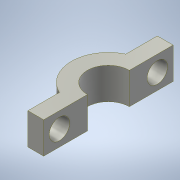
# Autodesk Inventor part: держатель
Saved by Autodesk Inventor 2021 (Build 250183000, 183)
## iProperties
Created: 2023-02-18
Part Number: держатель
Material: Типовые
Document SubType Name: Modeling
Designer: Tasya
Density: 1 g/cm^3
Appearance: Гладкий - слоновая кость
Author: Tasya
Autodesk Inventor part; units mm, degrees
ref_plane "YZ Plane" through (0, 0, 0) normal (1, 0, 0) x (0, 1, 0)
ref_plane "XZ Plane" through (0, 0, 0) normal (0, 1, 0) x (-1, 0, 0)
ref_plane "XY Plane" through (0, 0, 0) normal (0, 0, 1) x (1, 0, 0)
sketch "Эскиз1" plane through (0, 0, 0) normal (0, 1, 0) x (-1, 0, 0)
  line L0 (0, 12.3246) -> (0, 4)
  line L1 (0, 12.3246) -> (3, 12.3246)
  line L2 (3, 12.3246) -> (3, 6.3246)
  arc A0 (4, 0) -> (0, 4) centre (0, 0) ccw
  arc A1 (7, 0) -> (3, 6.3246) centre (0, 0) ccw
  line L3 (7, 0) -> (4, 0)
  line L4 (0, 0) -> (0, -3.8949) construction
  line L5 (0, 0) -> (4, 0) construction
  dimension "d0" = 4
  dimension "d1" = 7
  dimension "d2" = 6
  dimension "d3" = 3
  constraints: 12 end point, 4 point on circle, 3 horizontal, 2 centre point, 2 coincident, 2 collinear, 2 vertical, 1 perpendicular
  measures "d0" radius of A0
  measures "d1" radius of A1
  measures "d2" distance of L1.end L2.end
  measures "d3" distance of L0.start L1.end
extrude "Выдавливание1" add sketch "Эскиз1" along normal mid plane 6
sketch "Эскиз2" plane through (-3, -3, 12.3246) normal (-1, 0, 0) x (0, 0, 1)
  line L0 (0, 0) -> (0, 6) projected
  line L1 (-6, 6) -> (0, 6) projected
  line L2 (-6, 0) -> (-6, 6) projected
  line L3 (0, 0) -> (-6, 0) projected
  line L4 (0, 0) -> (-6, 6) construction
  line L5 (0, 6) -> (-8.3246, 6) construction
  line L6 (0, 6) -> (-6, 0) construction
  point P0 (-12.3246, 3)
  point P1 (-3, 3)
  constraints: 4 end point, 1 midpoint, 1 perpendicular
hole "Отверстие1" at (-3, 0, 9.3246) direction (1, 0, 0) diameter 3.9 end through all
mirror "Зеркальное отражение1" about plane through (0, 0, 0) normal (0, 0, 1) of "Выдавливание1", "Отверстие1"
